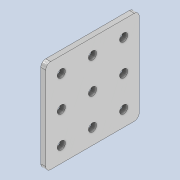
# Autodesk Inventor part: Generic 3x3 Corner Connecting Gusset
Saved by Autodesk Inventor 2022 (Build 260153000, 153)
## iProperties
Created: 2021-10-23
Part Number: Generic 3x3 Corner Connecting Gusset
Material: Generic
Document SubType Name: Modeling
Designer: Coy
Density: 1 g/cm^3
Appearance: Machined - Aluminum
Author: Coy
Autodesk Inventor part; units mm, degrees
ref_plane "YZ Plane" through (0, 0, 0) normal (1, 0, 0) x (0, 1, 0)
ref_plane "XZ Plane" through (0, 0, 0) normal (0, 1, 0) x (-1, 0, 0)
ref_plane "XY Plane" through (0, 0, 0) normal (0, 0, 1) x (1, 0, 0)
sketch "Sketch1" plane through (0, 0, 0) normal (1, 0, 0) x (0, 1, 0)
  line L0 (0, 0) -> (60, 0)
  line L1 (60, 0) -> (60, 60)
  line L2 (60, 60) -> (0, 60)
  line L3 (0, 60) -> (0, 0)
  line L4 (60, 60) -> (40, 60) construction
  line L5 (40, 60) -> (40, 40) construction
  line L6 (40, 40) -> (60, 40) construction
  line L7 (60, 40) -> (60, 60) construction
  line L8 (40, 40) -> (60, 40) construction
  line L9 (60, 40) -> (60, 20) construction
  line L10 (60, 20) -> (40, 20) construction
  line L11 (40, 20) -> (40, 40) construction
  line L12 (40, 20) -> (60, 20) construction
  line L13 (60, 20) -> (60, 0) construction
  line L14 (60, 0) -> (40, 0) construction
  line L15 (40, 0) -> (40, 20) construction
  line L16 (40, 20) -> (20, 20) construction
  line L17 (20, 20) -> (20, 0) construction
  line L18 (20, 0) -> (40, 0) construction
  line L19 (40, 0) -> (40, 20) construction
  line L20 (20, 20) -> (40, 20) construction
  line L21 (40, 20) -> (40, 40) construction
  line L22 (40, 40) -> (20, 40) construction
  line L23 (20, 40) -> (20, 20) construction
  line L24 (40, 40) -> (20, 40) construction
  line L25 (20, 40) -> (20, 60) construction
  line L26 (20, 60) -> (40, 60) construction
  line L27 (40, 60) -> (40, 40) construction
  line L28 (20, 60) -> (0, 60) construction
  line L29 (0, 60) -> (0, 40) construction
  line L30 (0, 40) -> (20, 40) construction
  line L31 (20, 40) -> (20, 60) construction
  line L32 (0, 40) -> (20, 40) construction
  line L33 (20, 40) -> (20, 20) construction
  line L34 (20, 20) -> (0, 20) construction
  line L35 (0, 20) -> (0, 40) construction
  line L36 (20, 20) -> (0, 20) construction
  line L37 (0, 20) -> (0, 0) construction
  line L38 (0, 0) -> (20, 0) construction
  line L39 (20, 0) -> (20, 20) construction
  line L40 (60, 10) -> (0, 10) construction
  line L41 (60, 30) -> (0, 30) construction
  line L42 (60, 50) -> (0, 50) construction
  line L43 (50, 60) -> (50, 0) construction
  line L44 (30, 60) -> (30, 0) construction
  line L45 (10, 60) -> (10, 0) construction
  circle A0 centre (50, 50) radius 2.6
  circle A1 centre (50, 30) radius 2.6
  circle A2 centre (50, 10) radius 2.6
  circle A3 centre (30, 10) radius 2.6
  circle A4 centre (30, 30) radius 2.6
  circle A5 centre (30, 50) radius 2.6
  circle A6 centre (10, 50) radius 2.6
  circle A7 centre (10, 30) radius 2.6
  circle A8 centre (10, 10) radius 2.6
  dimension "d0" = 60
  dimension "d1" = 60
  dimension "d2" = 20
  dimension "d3" = 20
  dimension "d4" = 20
  dimension "d5" = 20
  dimension "d6" = 20
  dimension "d7" = 20
  dimension "d8" = 20
  dimension "d9" = 20
  dimension "d10" = 5.2
  dimension "d11" = 5.2
  dimension "d12" = 5.2
  dimension "d13" = 5.2
  dimension "d14" = 5.2
  dimension "d15" = 5.2
  dimension "d16" = 5.2
  dimension "d17" = 5.2
  dimension "d18" = 5.2
  constraints: 92 end point, 20 parallel, 17 midpoint, 14 point on line, 10 horizontal, 10 perpendicular, 9 centre point
  measures "d0" distance of L2.end L1.end
  measures "d1" distance of L1.end L0.end
  measures "d2" distance of L6.end L5.end
  measures "d3" distance of L5.end L4.end
  measures "d4" distance of L9.end L10.end
  measures "d5" distance of L8.end L9.end
  measures "d6" distance of L0.end L14.end
  measures "d7" distance of L12.end L0.end
  measures "d8" distance of L18.end L17.end
  measures "d9" distance of L17.end L16.end
  measures "d10" diameter of A0
  measures "d11" diameter of A1
  measures "d12" diameter of A2
  measures "d13" diameter of A5
  measures "d14" diameter of A4
  measures "d15" diameter of A3
  measures "d16" diameter of A6
  measures "d17" diameter of A7
  measures "d18" diameter of A8
extrude "Extrusion1" add sketch "Sketch1" against normal blind 3.175
fillet "Fillet1" radius 3.175 4 edges at (-1.5875, 60, 60) (-1.5875, 0, 60) (-1.5875, 0, 0) (-1.5875, 60, 0)
equation "\"d11\" = d10"
equation "\"d12\" = d10"
equation "\"d13\" = d10"
equation "\"d14\" = d10"
equation "\"d15\" = d10"
equation "\"d16\" = d10"
equation "\"d17\" = d10"
equation "\"d18\" = d10"
body "Solid1"
